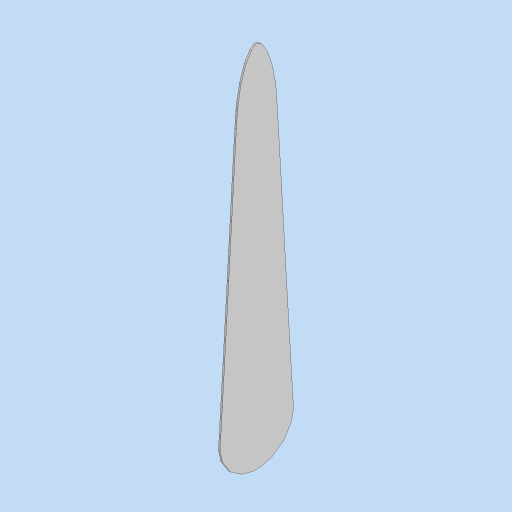
# Autodesk Inventor part: Sticker6
Saved by Autodesk Inventor 2024 (Build 280153000, 153)
## iProperties
Created: 2025-01-25
Part Number: Sticker6
Material: Generic
Document SubType Name: Modeling
Designer: Dmitry
Density: 1 g/cm^3
Appearance: Default
Author: Dmitry
Autodesk Inventor part; units mm, degrees
ref_plane "YZ Plane" through (0, 0, 0) normal (1, 0, 0) x (0, 1, 0)
ref_plane "XZ Plane" through (0, 0, 0) normal (0, 1, 0) x (-1, 0, 0)
ref_plane "XY Plane" through (0, 0, 0) normal (0, 0, 1) x (1, 0, 0)
sketch "Sketch1" plane through (0, 0, 0) normal (1, 0, 0) x (0, 1, 0)
  line L0 (-13.6199, 37.7174) -> (-13.6199, 37.7021)
  line L1 (-13.6199, 37.7021) -> (-13.6199, 37.664)
  line L2 (-13.6199, 37.664) -> (-13.6199, 37.6513)
  line L3 (-13.6199, 37.6513) -> (-13.6226, 37.0747)
  line L4 (-13.6226, 37.0747) -> (-13.1538, 35.3425)
  line L5 (-13.1538, 35.3425) -> (-11.8683, 33.4806)
  line L6 (-11.8683, 33.4806) -> (-9.9635, 32.2767)
  line L7 (-9.9635, 32.2767) -> (-8.2163, 31.8957)
  line L8 (-8.2163, 31.8957) -> (-7.643, 31.9312)
  line L9 (-7.643, 31.9312) -> (-6.3367, 32.0125)
  line L10 (-6.3367, 32.0125) -> (-2.4121, 32.2564)
  line L11 (-2.4121, 32.2564) -> (3.3634, 32.6094)
  line L12 (3.3634, 32.6094) -> (9.1619, 32.9625)
  line L13 (9.1619, 32.9625) -> (13.1363, 33.1987)
  line L14 (13.1363, 33.1987) -> (14.4621, 33.2774)
  line L15 (14.4621, 33.2774) -> (15.4583, 33.3359)
  line L16 (15.4583, 33.3359) -> (18.4512, 33.5111)
  line L17 (18.4512, 33.5111) -> (22.3554, 33.7423)
  line L18 (22.3554, 33.7423) -> (26.0527, 33.9607)
  line L19 (26.0527, 33.9607) -> (29.4232, 34.1614)
  line L20 (29.4232, 34.1614) -> (32.3475, 34.3417)
  line L21 (32.3475, 34.3417) -> (34.7054, 34.489)
  line L22 (34.7054, 34.489) -> (36.3755, 34.6008)
  line L23 (36.3755, 34.6008) -> (37.0247, 34.649)
  line L24 (37.0247, 34.649) -> (37.2396, 34.6719)
  line L25 (37.2396, 34.6719) -> (38.0554, 34.7633)
  line L26 (38.0554, 34.7633) -> (40.4847, 35.2307)
  line L27 (40.4847, 35.2307) -> (42.8482, 36.0029)
  line L28 (42.8482, 36.0029) -> (44.2921, 36.8715)
  line L29 (44.2921, 36.8715) -> (44.7829, 37.5142)
  line L30 (44.7829, 37.5142) -> (44.7829, 37.725)
  line L31 (44.7829, 37.725) -> (44.7829, 37.9383)
  line L32 (44.7829, 37.9383) -> (44.2921, 38.5708)
  line L33 (44.2921, 38.5708) -> (42.8482, 39.4395)
  line L34 (42.8482, 39.4395) -> (40.4847, 40.2091)
  line L35 (40.4847, 40.2091) -> (38.0554, 40.6739)
  line L36 (38.0554, 40.6739) -> (37.2396, 40.7654)
  line L37 (37.2396, 40.7654) -> (37.0247, 40.7908)
  line L38 (37.0247, 40.7908) -> (36.3755, 40.8365)
  line L39 (36.3755, 40.8365) -> (34.7042, 40.9508)
  line L40 (34.7042, 40.9508) -> (32.3448, 41.0981)
  line L41 (32.3448, 41.0981) -> (29.4177, 41.2784)
  line L42 (29.4177, 41.2784) -> (26.0445, 41.4791)
  line L43 (26.0445, 41.4791) -> (22.343, 41.6975)
  line L44 (22.343, 41.6975) -> (18.436, 41.9287)
  line L45 (18.436, 41.9287) -> (15.4418, 42.1039)
  line L46 (15.4418, 42.1039) -> (14.4441, 42.1624)
  line L47 (14.4441, 42.1624) -> (13.1197, 42.2386)
  line L48 (13.1197, 42.2386) -> (9.1482, 42.4773)
  line L49 (9.1482, 42.4773) -> (3.3547, 42.8278)
  line L50 (3.3547, 42.8278) -> (-2.4149, 43.1834)
  line L51 (-2.4149, 43.1834) -> (-6.3367, 43.4273)
  line L52 (-6.3367, 43.4273) -> (-7.643, 43.5086)
  line L53 (-7.643, 43.5086) -> (-8.2163, 43.5441)
  line L54 (-8.2163, 43.5441) -> (-9.9635, 43.1631)
  line L55 (-9.9635, 43.1631) -> (-11.8683, 41.9566)
  line L56 (-11.8683, 41.9566) -> (-13.1538, 40.0973)
  line L57 (-13.1538, 40.0973) -> (-13.6226, 38.3625)
  line L58 (-13.6226, 38.3625) -> (-13.6199, 37.7859)
  line L59 (-13.6199, 37.7859) -> (-13.6199, 37.7682)
  line L60 (-13.6199, 37.7682) -> (-13.6199, 37.7326)
  line L61 (-13.6199, 37.7326) -> (-13.6199, 37.7174)
  line L62 (-14.0082, 28.1898) -> (-14.295, 28.6115)
  line L63 (-14.295, 28.6115) -> (-14.4575, 28.8502)
  line L64 (-14.4575, 28.8502) -> (-14.5541, 28.9925)
  line L65 (-14.5541, 28.9925) -> (-15.0049, 29.5817)
  constraints: 132 end point
extrude "Extrusion27" add sketch "Sketch1" along normal blind 0.25
sketch "Sketch7" plane through (0, 0, 0) normal (-1, 0, 0) x (0, 0, 1)
  circle A0 centre (37.7743, -8.0049) radius 5.5
  circle A1 centre (37.7743, -8.0049) radius 0.5
  point P0 (0, 0)
  dimension "d91" = 11
  dimension "d92" = 1
  constraints: 2 centre point, 1 coincident
  measures "d91" diameter of A0
  measures "d92" diameter of A1
extrude "Extrusion30" [suppressed]
body "Solid6"
